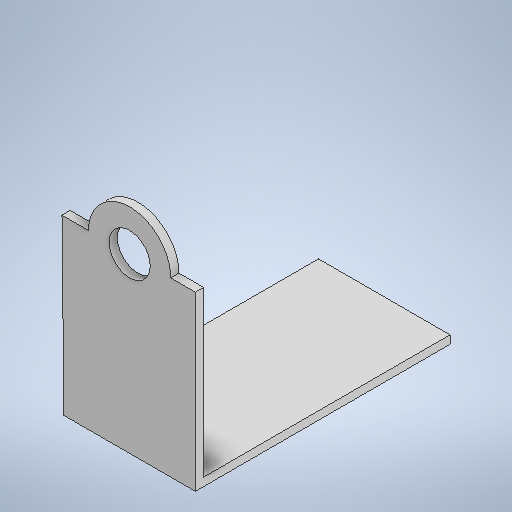
# Autodesk Inventor part: Resistencia_Lamina
Saved by Autodesk Inventor 2026 (Build 300175050, 175E)
## iProperties
Created: 2025-05-26
Part Number: Resistencia_Lamina
Material: Genérico
Document SubType Name: Modeling
Designer: alex
Density: 1 g/cm^3
Appearance: Valor por defecto
Author: alex
Autodesk Inventor part; units mm, degrees
ref_plane "YZ Plane" through (0, 0, 0) normal (1, 0, 0) x (0, 1, 0)
ref_plane "XZ Plane" through (0, 0, 0) normal (0, 1, 0) x (-1, 0, 0)
ref_plane "XY Plane" through (0, 0, 0) normal (0, 0, 1) x (1, 0, 0)
sketch "Boceto1" plane through (0, 0, 0) normal (0, 0, 1) x (1, 0, 0)
  circle A0 centre (0, 0) radius 2.5
  line L0 (5, 0) -> (8, 0)
  line L1 (8, 0) -> (8, -21)
  line L2 (8, -21) -> (-5, -21)
  line L3 (-5, -21) -> (-8, -21)
  line L4 (-8, -21) -> (-8.2375, 0)
  line L5 (-8.2375, 0) -> (-5, 0)
  arc A1 (5, 0) -> (-5, 0) centre (0, 0) ccw
  dimension "d0" = 5
  dimension "d2" = 3
  dimension "d3" = 21
  dimension "d4" = 3
  constraints: 12 end point, 3 point on line, 2 centre point, 2 perpendicular, 2 point on circle, 1 coincident, 1 horizontal
  measures "d0" diameter of A0
  measures "d2" distance of L0.start L0.end
  measures "d3" distance of L0.end L1.end
  measures "d4" distance of L2.end L3.end
extrude "Extrusión1" add sketch "Boceto1" along normal blind 1
sketch "Boceto2" plane through (0, 0, 0) normal (0, 0, -1) x (-1, 0, 0)
  line L0 (8, -21) -> (-8, -21) projected
  line L1 (8.2375, 0) -> (8, -21) projected
  line L2 (-8, -21) -> (8.0113, -21)
  line L3 (8.0113, -21) -> (8.0113, -20)
  line L4 (8.0113, -20) -> (-8, -20)
  line L5 (-8, -20) -> (-8, -21)
  point P0 (0, 0)
  dimension "d7" = 1
  constraints: 8 end point, 2 parallel, 1 horizontal, 1 perpendicular, 1 point on line
  measures "d7" distance of L3.end L2.end
extrude "Extrusión2" add sketch "Boceto2" along normal blind 30
